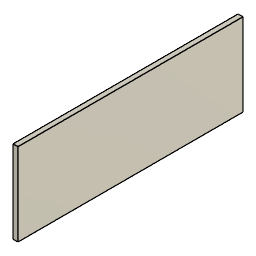
divider (Autodesk Fusion 360 design; units mm, degrees)
part number: 2026-08-18-20-59-33-803
Autodesk Fusion 360 part; units mm, degrees
sketch "Sketch1" plane through (0, 0, 0) normal (0, 0, 1) x (1, 0, 0)
  line L0 (0, 0) -> (2.4, 0)
  line L1 (2.4, 0) -> (2.4, 109)
  line L2 (2.4, 109) -> (0, 109)
  line L3 (0, 109) -> (0, 0)
extrude "Extrude1" add sketch "Sketch1" along normal blind 40
named bodies: "Тело"
